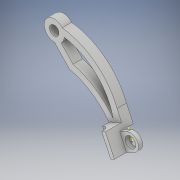
# Autodesk Inventor part: Beta_arm
Saved by Autodesk Inventor 2018 (Build 220112000, 112)
## iProperties
Created: 2017-10-02
Part Number: Beta_arm
Material: Generic
Document SubType Name: Modeling
Designer: rheal
Density: 1 g/cm^3
Appearance: Default
Author: rheal
Autodesk Inventor part; units mm, degrees
ref_plane "YZ Plane" through (0, 0, 0) normal (1, 0, 0) x (0, 1, 0)
ref_plane "XZ Plane" through (0, 0, 0) normal (0, 1, 0) x (-1, 0, 0)
sketch "Sketch1" plane through (0, 0, 0) normal (0, 0, 1) x (1, 0, 0)
  arc A0 (-3.4091, 18.1463) -> (-44.1177, 49.6528) centre (-50, 0) ccw
  arc A1 (-4.5455, -2.083) -> (-38.7191, 25.7979) centre (-50, -22.9129) ccw
  arc A2 (-6.2101, 10.3653) -> (-42.5261, 44.375) centre (-50, 0) ccw
  line L0 (5, 0) -> (-3.4091, 18.1463)
  arc A3 (-4.5455, -2.083) -> (5, 0) centre (0, 0) ccw
  line L1 (-50, 32.0871) -> (-50, 50) construction
  line L2 (-50, 37.7239) -> (-44.3975, 31.801)
  line L3 (-44.8461, 39.5514) -> (-40.7651, 35.237)
  line L4 (-44.3975, 31.801) -> (-38.7191, 25.7979)
  line L5 (-40.7651, 35.237) -> (-36.0957, 30.3006)
  arc A4 (-6.2101, 10.3653) -> (-36.0957, 30.3006) centre (-50, -22.9129) ccw
  circle A5 centre (-50, 45) radius 3.5
  arc A6 (-44.8461, 39.5514) -> (-42.5261, 44.375) centre (-50, 45) ccw
  arc A7 (-44.1177, 49.6528) -> (-49.7909, 37.5029) centre (-50, 45) ccw
  point P0 (19.05, 139.7)
  dimension "d65" = 5
  dimension "d66" = 20
  dimension "d74" = 5
  dimension "d75" = 7
  constraints: 14 point on circle, 12 end point, 8 centre point, 2 coincident, 2 parallel, 2 point on line, 1 vertical
  measures "d65" radial gap between concentric circles of A0 A2
  measures "d66" distance of L0.end L0.start
  measures "d74" distance between parallel lines of L2 L3
  measures "d75" diameter of A5
extrude "Extrusion12" add sketch "Sketch1" along normal blind 7
sketch "Sketch16" plane through (0, 0, 7) normal (0, 0, 1) x (1, 0, 0)
  point P0 (0, 0)
sketch "Sketch19" plane through (0, 0, 0) normal (0, 0, -1) x (-1, 0, 0)
  circle A0 centre (0, 0) radius 1.5
  dimension "d101" = 3
  constraints: 1 centre point, 1 coincident
  measures "d101" diameter of A0
extrude "Extrusion16" cut sketch "Sketch19" against normal blind 10
sketch "Sketch24" plane through (0, 0, 0) normal (0, 0, -1) x (-1, 0, 0)
  circle A0 centre (0, 0) radius 1.5 projected
  circle A1 centre (0, 0) radius 7.5
  dimension "d115" = 15
  constraints: 1 centre point, 1 coincident
  measures "d115" diameter of A1
extrude "Extrusion19" cut sketch "Sketch24" against normal blind 4
ref_plane "Work Plane9" through (5, 0, 7) normal (-0.4204545, 0.9073136, 0) x (-0.9073136, -0.4204545, 0)
sketch "Sketch25" plane through (0, 0, 7) normal (0, 0, 1) x (1, 0, 0)
  point P0 (0, 0)
sketch "Sketch26" plane through (5, 0, 7) normal (-0.4204545, 0.9073136, 0) x (-0.9073136, -0.4204545, 0)
  point P0 (4.5366, -7)
sketch "Sketch27" plane through (5, 0, 7) normal (-0.4204545, 0.9073136, 0) x (-0.9073136, -0.4204545, 0)
  line L0 (0, -7) -> (0, 0) projected
  line L1 (0, 0) -> (0, 12)
  line L2 (0, 12) -> (3, 12)
  line L3 (0, 0) -> (9.5, 0)
  line L4 (24.5467, 0) -> (5.8129, 0) projected
  line L5 (9.5, 0) -> (9.5, 5.5)
  arc A0 (3, 12) -> (9.5, 5.5) centre (8.9772, 11.4772) ccw
  point P0 (4.5366, -7)
  dimension "d118" = 12
  dimension "d119" = 3
  dimension "d120" = 9.5
  dimension "d121" = 5.5
  dimension "d122" = 6
  constraints: 8 end point, 2 perpendicular, 2 point on circle, 1 centre point, 1 point on line, 1 vertical
  measures "d118" distance of L0.end L1.end
  measures "d119" distance of L1.end L2.end
  measures "d120" distance of L0.end L3.end
  measures "d121" distance of L3.end L5.end
  measures "d122" radius of A0
extrude "Extrusion20" add sketch "Sketch27" along normal blind 12 and the other way blind 3.85
sketch "Sketch30" plane through (0, 0, 4) normal (0, 0, -1) x (-1, 0, 0)
  line L0 (0, 0) -> (-4.9989, 2.3165)
  line L1 (-5, 0) -> (-1.605, 7.3263) projected
  constraints: 2 end point, 1 perpendicular
sketch "Sketch31" plane through (-3.4091, 18.1463, 7) normal (0.9073136, 0.4204545, 0) x (0, 0, -1)
  line L0 (-15.8, -20) -> (10.8, -20) projected
  line L1 (3, -17.8765) -> (3, -12.5529) projected
  line L2 (3, -17.8765) -> (3, -11.8765)
  line L3 (3, -11.8765) -> (0, -11.8765)
  line L4 (3, -17.8765) -> (0, -17.8765) projected
  line L5 (3, -17.8765) -> (3, -23.8765)
  line L6 (3, -17.8765) -> (3, -22.8977) projected
  line L7 (0, -11.8765) -> (-3, -11.8765)
  line L8 (-3, -11.8765) -> (-3, -23.8765)
  line L9 (-3, -23.8765) -> (0, -23.8765)
  line L10 (0, -23.8765) -> (0, -11.8765)
  point P0 (7, -17.8977)
  point P1 (3, -20)
  dimension "d129" = 6
  dimension "d130" = 3
  dimension "d131" = 6
  dimension "d132" = 3
  constraints: 14 end point, 2 collinear, 2 parallel, 2 perpendicular, 1 horizontal
  measures "d129" distance of L1.start L2.end
  measures "d130" distance of L2.end L3.end
  measures "d131" distance of L1.start L5.end
  measures "d132" distance of L9.end L8.end
extrude "Extrusion21" add sketch "Sketch31" along normal blind 12 contours L8 L7 L10 L0 | L0 L10 L9 L8
sketch "Sketch32" plane through (6.6188, -3.4932, 10) normal (0, 0, 1) x (0.9073136, 0.4204545, 0)
  line L0 (0, 11.9735) -> (0, 3.85) projected
  line L1 (0, 6.0521) -> (5.9995, 5.974) construction
  circle A0 centre (5.9995, 5.974) radius 4
  line L2 (6, 11.9735) -> (6, -0.0265) construction
  arc A1 (0, 6.0005) -> (0, 5.9475) centre (5.9995, 5.974) ccw
  line L3 (6, -0.0265) -> (12, -0.0265)
  point P0 (-4.5366, 5.9523)
  point P1 (12, 11.9735)
  dimension "d139" = 6
  dimension "d140" = 8
  constraints: 6 end point, 4 point on line, 2 centre point, 2 coincident, 2 point on circle
  measures "d139" distance of L1.start L1.end
  measures "d140" diameter of A0
extrude "Extrusion22" cut sketch "Sketch32" against normal blind 3
fillet "Fillet5" radius 6 2 edges at (12.4722, 12.416, 8.5) (17.5177, 1.5283, 8.5)
body "Solid1"
